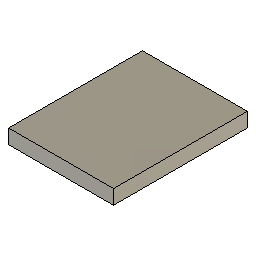
battery (Autodesk Fusion 360 design; units mm, degrees)
part number: 2025-08-31-09-58-57-639
Autodesk Fusion 360 part; units mm, degrees
sketch "Sketch1" plane through (0, 0, 0) normal (0, 0, 1) x (1, 0, 0)
  line L0 (-14.5, -18.5) -> (14.5, -18.5)
  line L1 (14.5, -18.5) -> (14.5, 18.5)
  line L2 (14.5, 18.5) -> (-14.5, 18.5)
  line L3 (-14.5, 18.5) -> (-14.5, -18.5)
  line L4 (-14.5, 18.5) -> (14.5, -18.5) construction
  dimension "d1" = 29
  dimension "d2" = 37
  constraint horizontal L0
  constraint vertical L1
  constraint horizontal L2
  constraint vertical L3
  constraint midpoint origin L4
  measures "d1" distance of L0.start L0.end
  measures "d2" distance of L0.start L2.end
extrude "Extrude1" add sketch "Sketch1" along normal blind 4
